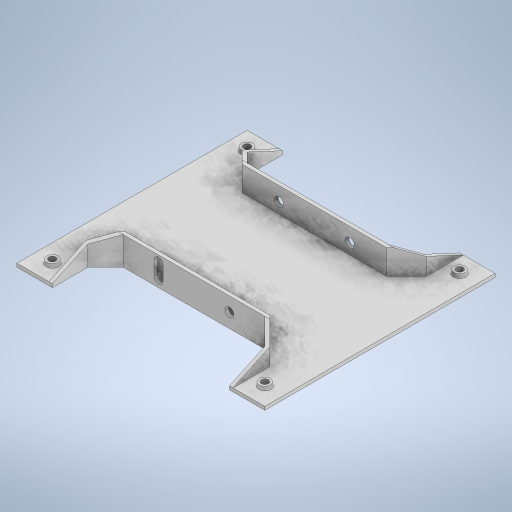
# Autodesk Inventor part: ChairBaseBracket
Saved by Autodesk Inventor 2023 (Build 270158030, 158C)
## iProperties
Created: 2023-03-04
Part Number: ChairBaseBracket
Material: Generic
Document SubType Name: Modeling
Designer: mpino
Density: 1 g/cm^3
Appearance: Default
Author: mpino
Autodesk Inventor part; units mm, degrees
ref_plane "YZ Plane" through (0, 0, 0) normal (1, 0, 0) x (0, 1, 0)
ref_plane "XZ Plane" through (0, 0, 0) normal (0, 1, 0) x (-1, 0, 0)
ref_plane "XY Plane" through (0, 0, 0) normal (0, 0, 1) x (1, 0, 0)
sketch "Sketch1" plane through (0, 0, 0) normal (0, 1, 0) x (-1, 0, 0)
  line L0 (0, 0) -> (0, -165.1)
  line L1 (0, -165.1) -> (-177.8, -165.1)
  line L2 (-177.8, -165.1) -> (-177.8, 0)
  line L3 (-177.8, 0) -> (0, 0)
  line L4 (0, 0) -> (-25.4, 0)
  line L5 (-177.8, 0) -> (-152.4, 0)
  line L6 (0, -165.1) -> (-25.4, -165.1)
  line L7 (-177.8, -165.1) -> (-152.4, -165.1)
  line L8 (-152.4, 0) -> (-152.4, -25.4)
  line L9 (-152.4, -165.1) -> (-152.4, -139.7)
  line L10 (-25.4, 0) -> (-25.4, -25.4)
  line L11 (-25.4, -165.1) -> (-25.4, -139.7)
  line L12 (-38.1, -38.1) -> (-139.7, -38.1)
  line L13 (-25.4, -25.4) -> (-38.1, -38.1)
  line L14 (-25.4, -25.4) -> (-7.439488, -25.4) construction
  line L15 (-152.4, -25.4) -> (-139.7, -38.1)
  line L16 (-177.8, -82.55) -> (0, -82.55)
  line L17 (-152.4, -165.1) -> (-152.4, -139.7)
  line L18 (-25.4, -165.1) -> (-25.4, -139.7)
  line L19 (-38.1, -127) -> (-139.7, -127)
  line L20 (-25.4, -139.7) -> (-38.1, -127)
  line L21 (-152.4, -139.7) -> (-139.7, -127)
  dimension "d1" = 165.1
  dimension "d2" = 177.8
  dimension "d3" = 25.4
  dimension "d4" = 25.4
  dimension "d6" = 25.4
  dimension "d7" = 25.4
  dimension "d10" = 25.4
  dimension "d11" = 25.4
  dimension "d12" = 25.4
  dimension "d13" = 25.4
  dimension "d16" = 101.6
  dimension "d17" = 135
  dimension "d18" = 135
  constraints: 46 end point, 5 vertical, 4 point on line, 3 perpendicular, 2 horizontal, 2 midpoint, 2 symmetric about line, 1 equal length
  measures "d1" distance of L0.start L0.end
  measures "d2" distance of L0.end L1.end
  measures "d3" distance of L0.start L4.end
  measures "d4" distance of L2.end L5.end
  measures "d6" distance of L0.end L6.end
  measures "d7" distance of L1.end L7.end
  measures "d10" distance of L5.end L8.end
  measures "d11" distance of L7.end L9.end
  measures "d12" distance of L4.end L10.end
  measures "d13" distance of L6.end L11.end
  measures "d16" distance of L12.start L12.end
  measures "d17" angle of L13 L14
  measures "d18" angle of L15 L8
extrude "Extrusion1" add sketch "Sketch1" along normal blind 2.54 contours L0 L16 L2 L3 L8 L15 L12 L13 L10 | L0 L1 L11 L20 L19 L21 L9 L2 L16
sketch "Sketch2" plane through (0, 2.54, 0) normal (0, 1, 0) x (1, 0, 0)
  line L0 (25.4, 139.7) -> (25.4, 165.1)
  line L1 (25.4, 165.1) -> (0, 165.1)
  line L2 (0, 165.1) -> (0, 0)
  line L3 (0, 0) -> (25.4, 0)
  line L4 (25.4, 0) -> (25.4, 25.4)
  line L5 (25.4, 25.4) -> (38.1, 38.1)
  line L6 (38.1, 38.1) -> (139.7, 38.1)
  line L7 (139.7, 38.1) -> (152.4, 25.4)
  line L8 (152.4, 25.4) -> (152.4, 0)
  line L9 (152.4, 0) -> (177.8, 0)
  line L10 (177.8, 0) -> (177.8, 165.1)
  line L11 (177.8, 165.1) -> (152.4, 165.1)
  line L12 (152.4, 165.1) -> (152.4, 139.7)
  line L13 (152.4, 139.7) -> (139.7, 127)
  line L14 (139.7, 127) -> (38.1, 127)
  line L15 (38.1, 127) -> (25.4, 139.7)
  line L16 (2.54, 2.54) -> (2.54, 162.56)
  line L17 (2.54, 162.56) -> (22.86, 162.56)
  line L18 (22.86, 162.56) -> (22.86, 138.647898)
  line L19 (22.86, 138.647898) -> (37.047898, 124.46)
  line L20 (37.047898, 124.46) -> (140.752102, 124.46)
  line L21 (140.752102, 124.46) -> (154.94, 138.647898)
  line L22 (154.94, 138.647898) -> (154.94, 162.56)
  line L23 (154.94, 162.56) -> (175.26, 162.56)
  line L24 (175.26, 162.56) -> (175.26, 2.54)
  line L25 (175.26, 2.54) -> (154.94, 2.54)
  line L26 (154.94, 2.54) -> (154.94, 26.452102)
  line L27 (154.94, 26.452102) -> (140.752102, 40.64)
  line L28 (140.752102, 40.64) -> (37.047898, 40.64)
  line L29 (37.047898, 40.64) -> (22.86, 26.452102)
  line L30 (22.86, 26.452102) -> (22.86, 2.54)
  line L31 (22.86, 2.54) -> (2.54, 2.54)
  line L32 (22.86, 2.54) -> (22.86, 0)
  line L33 (154.94, 2.54) -> (154.94, 0)
  line L34 (154.94, 162.56) -> (154.94, 165.1)
  line L35 (22.86, 162.56) -> (22.86, 165.1)
  dimension "d21" = 2.54
  constraints: 40 end point, 4 point on line, 3 vertical, 1 perpendicular, 15 other
  measures "d21" distance between parallel lines of L2 L16
extrude "Extrusion2" add sketch "Sketch2" along normal blind 17.78 contours L15 L14 L13 L12 L11 L34 L22 L21 L20 L19 L18 L35 L1 L0 | L32 L30 L29 L28 L27 L26 L33 L9 L8 L7 L6 L5 L4 L3
sketch "Sketch3" plane through (154.94, 2.54, 0) normal (1, 0, 0) x (0, 0, -1)
  line L0 (165.1, 0) -> (0, 0)
  line L1 (26.452102, 0) -> (26.452102, 17.78)
  line L2 (0, 17.78) -> (0, 0)
  line L3 (38.1, -2.54) -> (38.1, 17.78)
  line L4 (0, 0) -> (38.1, 17.78)
  line L5 (38.1, 17.78) -> (0, 17.78)
  line L6 (165.1, -2.54) -> (165.1, 17.78)
  line L7 (165.1, 0) -> (165.1, 17.78)
  line L8 (127, -2.54) -> (127, 17.78)
  line L9 (165.1, 17.78) -> (127, 17.78)
  line L10 (127, 17.78) -> (165.1, 0)
  point P0 (0, -2.54)
  dimension "d24" = 17.78
  constraints: 12 end point, 2 perpendicular, 1 collinear
  measures "d24" distance of L2.start L0.end
extrude "Extrusion3" cut sketch "Sketch3" against normal blind 132.08 contours L2 L5 L1 L4 | L1 L5 L4 | L10 L9 L6
sketch "Sketch4" plane through (0, 2.54, 0) normal (0, 1, 0) x (1, 0, 0)
  line L0 (0, 0) -> (0, 25.4)
  line L1 (0, 165.1) -> (0, 0) projected
  line L2 (0, 25.4) -> (25.4, 25.4)
  line L3 (0, 0) -> (25.4, 0) projected
  line L4 (25.4, 25.4) -> (0, 0)
  line L5 (0, 25.4) -> (25.4, 0)
  circle A0 centre (12.7, 12.7) radius 4.445
  dimension "d27" = 25.4
  dimension "d28" = 25.4
  dimension "d29" = 8.89
  constraints: 8 end point, 1 centre point, 1 midpoint, 1 perpendicular, 1 point on line
  measures "d27" distance of L0.start L0.end
  measures "d28" distance of L0.end L2.end
  measures "d29" diameter of A0
sketch "Sketch4 outline for Extrusion4" plane through (0, 2.54, 0) normal (0, 1, 0) x (1, 0, 0)
  circle A0 centre (12.7, 12.7) radius 4.445
extrude "Extrusion4" add sketch "Sketch4 outline for Extrusion4" along normal blind 2.54 draft -10
sketch "Sketch5" plane through (12.7, 5.08, -12.7) normal (0, 1, 0) x (1, 0, 0)
  circle A0 centre (0, 0) radius 3.997129
  line L0 (0, -3.997129) -> (0, 3.997129)
  line L1 (3.997129, 0) -> (-3.997129, 0)
  point P0 (-12.7, -12.7)
  dimension "d32" = 7.99426
  dimension "d33" = 7.99426
  constraints: 4 end point, 4 point on circle, 1 perpendicular, 1 vertical
  measures "d32" distance of L0.start L0.end
  measures "d33" distance of L1.start L1.end
hole "Hole1" at (12.7, 5.08, -12.7) direction (0, -1, 0) diameter 4.9784 end through all thread size "1/4-20 UNC" class "2B" standard "ANSI Unified Screw Threads"
pattern_linear "Rectangular Pattern1" count 2 spacing 139.7 along (0, 0, -1) count 2 spacing 152.4 along (1, 0, 0) of "Hole1", "Extrusion4"
sketch "Sketch6" plane through (139.7, 0, -127) normal (0, 0, -1) x (-1, 0, 0)
  line L0 (101.6, 0) -> (101.6, 20.32) projected
  line L1 (0, 0) -> (0, 20.32) projected
  line L2 (101.6, 0) -> (0, 20.32)
  line L3 (0, 20.32) -> (0, 0)
  line L4 (0, 0) -> (101.6, 20.32)
  line L5 (50.8, 10.16) -> (76.2, 10.16)
  line L6 (50.8, 10.16) -> (25.4, 10.16)
  circle A0 centre (76.2, 10.16) radius 3.175
  circle A1 centre (25.4, 10.16) radius 3.175
  point P0 (139.7, 0)
  dimension "d48" = 101.6
  dimension "d49" = 22.6199
  dimension "d51" = 25.4
  dimension "d52" = 25.4
  dimension "d53" = 6.35
  dimension "d54" = 6.35
  constraints: 10 end point, 2 centre point, 2 coincident, 1 collinear, 1 horizontal, 1 midpoint, 1 point on line
  measures "d48" horizontal distance of L1.start L4.end
  measures "d49" angle of L2 L4
  measures "d51" distance of L5.start L5.end
  measures "d52" distance of L5.start L6.end
  measures "d53" diameter of A0
  measures "d54" diameter of A1
extrude "Extrusion5" cut sketch "Sketch6" against normal blind 88.9 contours A0 | A1
sketch "Sketch7" plane through (38.1, 0, -38.1) normal (0, 0, 1) x (1, 0, 0)
  circle A0 centre (25.4, 10.16) radius 3.175 projected
  line L0 (25.4, 10.16) -> (22.225, 10.16)
  line L1 (22.225, 10.16) -> (22.225, 5.715)
  line L2 (22.225, 5.715) -> (25.4, 5.715)
  circle A1 centre (25.4, 5.715) radius 3.175
  line L3 (28.575, 5.715) -> (28.575, 15.875)
  line L4 (28.575, 15.875) -> (25.4, 15.875)
  circle A2 centre (25.4, 15.875) radius 3.175
  line L5 (22.225, 10.16) -> (22.225, 15.875)
  line L6 (25.4, 0) -> (25.4, 2.54)
  point P0 (-38.1, 0)
  point P1 (22.225, 13.0175)
  dimension "d58" = 6.35
  dimension "d57" = 4.445
  dimension "d60" = 6.35
  dimension "d61" = 6.35
  dimension "d62" = 5.715
  dimension "d63" = 2.54
  dimension "d64" = 3.175
  dimension "d65" = 13.335
  constraints: 14 end point, 4 vertical, 2 coincident, 2 horizontal, 2 point on circle, 1 centre point, 1 horizontal alignment, 1 midpoint, 1 perpendicular, 1 tangent, 4 other
  measures "d57" distance of L0.end L1.end
  measures "d60" diameter of A2
  measures "d61" distance from line of point (22.225, 13.017) L3
  measures "d62" distance of L4.end L0.start
  measures "d63" distance of L6.start L6.end
  measures "d64" distance between parallel lines of L6 L3
  measures "d65" distance from line of L6.end L4
extrude "Extrusion6" cut sketch "Sketch7" against normal blind 2.54
body "Solid1"
